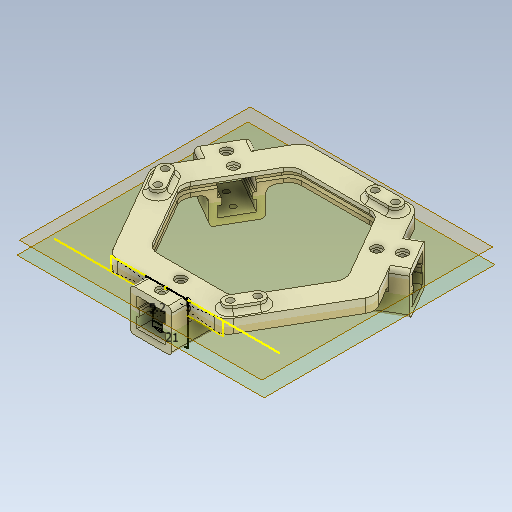
# Autodesk Inventor part: upper_board_mount
Saved by Autodesk Inventor 2021 (Build 250183000, 183)
## iProperties
Created: 2021-01-25
Part Number: upper_board_mount
Material: PC/ABS 플라스틱
Document SubType Name: Modeling
Designer: leejun
Density: 0.357273 g/cm^3
Appearance: 매끄러움 - 물푸레나무색
Author: leejun
Autodesk Inventor part; units mm, degrees
ref_plane "YZ Plane" through (0, 0, 0) normal (1, 0, 0) x (0, 1, 0)
ref_plane "XZ Plane" through (0, 0, 0) normal (0, 1, 0) x (-1, 0, 0)
ref_plane "XY Plane" through (0, 0, 0) normal (0, 0, 1) x (1, 0, 0)
sketch "스케치1" plane through (0, 0, 0) normal (0, 1, 0) x (-1, 0, 0)
  line L0 (128.6603, -74.282) -> (42.8868, -74.282) construction
  line L1 (-128.6603, -74.282) -> (0, 148.5641) construction
  line L2 (0, 148.5641) -> (128.6603, -74.282) construction
  line L3 (40, -69.282) -> (-40, -69.282) construction
  line L4 (-40, -69.282) -> (-40, -56.582) construction
  line L5 (-40, -56.582) -> (40, -56.582) construction
  line L6 (40, -56.582) -> (40, -69.282) construction
  line L7 (-80, 0) -> (-40, 69.282) construction
  line L8 (-40, 69.282) -> (-29.0015, 62.932) construction
  line L9 (-29.0015, 62.932) -> (-69.0015, -6.35) construction
  line L10 (-69.0015, -6.35) -> (-80, 0) construction
  line L11 (40, 69.282) -> (29.0015, 62.932) construction
  line L12 (29.0015, 62.932) -> (69.0015, -6.35) construction
  line L13 (69.0015, -6.35) -> (80, 0) construction
  line L14 (80, 0) -> (40, 69.282) construction
  line L15 (85.7735, 0) -> (42.8868, -74.282) construction
  line L16 (-42.8868, -74.282) -> (-85.7735, 0) construction
  line L17 (42.8868, 74.282) -> (-42.8868, 74.282) construction
  circle A0 centre (72.0007, 1.1551) radius 6.35 construction
  circle A1 centre (64.5007, 14.1455) radius 6.35 construction
  circle A2 centre (-35, -62.932) radius 6.35 construction
  circle A3 centre (-20, -62.932) radius 6.35 construction
  circle A4 centre (-37.0007, 61.7769) radius 6.35 construction
  circle A5 centre (-44.5007, 48.7865) radius 6.35 construction
  circle A6 centre (72.0007, 1.1551) radius 2.65
  circle A7 centre (64.5007, 14.1455) radius 2.65
  circle A8 centre (-20, -62.932) radius 2.65
  circle A9 centre (-35, -62.932) radius 2.65
  circle A10 centre (-44.5007, 48.7865) radius 2.65
  circle A11 centre (-37.0007, 61.7769) radius 2.65
  line L18 (40, -56.582) -> (-40, -69.282) construction
  line L19 (-40, -56.582) -> (40, -69.282) construction
  line L20 (69.0015, -6.35) -> (40, 69.282) construction
  line L21 (80, 0) -> (29.0015, 62.932) construction
  line L22 (-29.0015, 62.932) -> (-80, 0) construction
  line L23 (-69.0015, -6.35) -> (-40, 69.282) construction
  line L24 (72.0007, 1.1551) -> (64.5007, 14.1455) construction
  line L25 (-20, -62.932) -> (-35, -62.932) construction
  line L26 (-37.0007, 61.7769) -> (-44.5007, 48.7865) construction
  circle A12 centre (35, -62.932) radius 2.15 construction
  circle A13 centre (20, -62.932) radius 2.15 construction
  circle A14 centre (44.5007, 48.7865) radius 2.15 construction
  circle A15 centre (37.0007, 61.7769) radius 2.15 construction
  circle A16 centre (-72.0007, 1.1551) radius 2.15 construction
  circle A17 centre (-64.5007, 14.1455) radius 2.15 construction
  line L27 (42.8868, -74.282) -> (-42.8868, -74.282) construction
  line L28 (-42.8868, -74.282) -> (-128.6603, -74.282) construction
  line L29 (0, -62.932) -> (-54.5007, 31.466) construction
  line L30 (-54.5007, 31.466) -> (54.5007, 31.466) construction
  line L31 (54.5007, 31.466) -> (0, -62.932) construction
  line L32 (68.844, -27.6227) -> (58.344, -45.8093)
  line L33 (58.344, -45.8093) -> (40.1575, -35.3093)
  line L34 (40.1575, -35.3093) -> (50.6575, -17.1227)
  line L35 (50.6575, -17.1227) -> (68.844, -27.6227)
  line L36 (10.5, 73.432) -> (-10.5, 73.432)
  line L37 (-10.5, 73.432) -> (-10.5, 52.432)
  line L38 (-10.5, 52.432) -> (10.5, 52.432)
  line L39 (10.5, 52.432) -> (10.5, 73.432)
  line L40 (-58.344, -45.8093) -> (-68.844, -27.6227)
  line L41 (-68.844, -27.6227) -> (-50.6575, -17.1227)
  line L42 (-50.6575, -17.1227) -> (-40.1575, -35.3093)
  line L43 (-40.1575, -35.3093) -> (-58.344, -45.8093)
  line L44 (45.4075, -26.216) -> (-45.4075, -26.216) construction
  line L45 (-45.4075, -26.216) -> (0, 52.432) construction
  line L46 (0, 52.432) -> (45.4075, -26.216) construction
  line L47 (61.8712, 0) -> (30.9356, -53.582)
  line L48 (30.9356, -53.582) -> (-30.9356, -53.582)
  line L49 (-30.9356, -53.582) -> (-61.8712, 0)
  line L50 (-61.8712, 0) -> (-30.9356, 53.582)
  line L51 (-30.9356, 53.582) -> (30.9356, 53.582)
  line L52 (30.9356, 53.582) -> (61.8712, 0)
  line L53 (83.4641, 0) -> (41.7321, -72.282)
  line L54 (41.7321, -72.282) -> (-41.7321, -72.282)
  line L55 (-41.7321, -72.282) -> (-83.4641, 0)
  line L56 (-83.4641, 0) -> (-41.7321, 72.282)
  line L57 (-41.7321, 72.282) -> (41.7321, 72.282)
  line L58 (41.7321, 72.282) -> (83.4641, 0)
  line L59 (68.844, -27.6227) -> (40.1575, -35.3093) construction
  line L60 (58.344, -45.8093) -> (50.6575, -17.1227) construction
  circle A18 centre (54.5007, -31.466) radius 9.35 construction
  line L61 (71.0668, -21.4727) -> (73.9536, -26.4727)
  line L62 (73.9536, -26.4727) -> (59.9029, -50.8093)
  line L63 (59.9029, -50.8093) -> (54.1293, -50.8093)
  line L64 (54.8721, -12.1227) -> (49.0986, -12.1227)
  line L65 (49.0986, -12.1227) -> (35.0479, -36.4593)
  line L66 (35.0479, -36.4593) -> (37.9347, -41.4593)
  line L67 (16.9375, 53.582) -> (14.0507, 48.582)
  line L68 (14.0507, 48.582) -> (-14.0507, 48.582)
  line L69 (-14.0507, 48.582) -> (-16.9375, 53.582)
  line L70 (16.9375, 72.282) -> (14.0507, 77.282)
  line L71 (14.0507, 77.282) -> (-14.0507, 77.282)
  line L72 (-14.0507, 77.282) -> (-16.9375, 72.282)
  line L73 (-37.9347, -41.4593) -> (-35.0479, -36.4593)
  line L74 (-35.0479, -36.4593) -> (-49.0986, -12.1227)
  line L75 (-49.0986, -12.1227) -> (-54.8721, -12.1227)
  line L76 (-71.0668, -21.4727) -> (-73.9536, -26.4727)
  line L77 (-73.9536, -26.4727) -> (-59.9029, -50.8093)
  line L78 (-59.9029, -50.8093) -> (-54.1293, -50.8093)
  line L79 (42.8868, 74.282) -> (40, 69.282) construction
  line L80 (80, 0) -> (85.7735, 0) construction
  point P0 (0, 0)
  point P1 (0, 0)
  point P2 (0, 0)
  point P3 (0, 0)
  point P4 (0, 0)
  point P5 (0, 0)
  point P6 (0, 0)
  dimension "d1" = 12.7
  dimension "d12" = 80
  dimension "d13" = 5.3
  dimension "d14" = 5
  dimension "d15" = 20
  dimension "d16" = 5
  dimension "d17" = 20
  dimension "d18" = 5
  dimension "d19" = 20
  dimension "d79" = 4.3
  dimension "d80" = 5
  dimension "d81" = 15
  dimension "d82" = 5
  dimension "d83" = 15
  dimension "d84" = 5
  dimension "d85" = 15
  dimension "d86" = 5
  dimension "d88" = 21
  dimension "d89" = 3
  dimension "d90" = 3
  dimension "d92" = 5
  dimension "d93" = 5
  dimension "d95" = 5
  dimension "d96" = 5
  dimension "d97" = 5
  dimension "d98" = 5
  dimension "d99" = 5
  dimension "d100" = 5
  dimension "d101" = 5
  dimension "d102" = 5
  dimension "d103" = 5
  dimension "d104" = 5
  dimension "d105" = 5
  dimension "d106" = 5
  dimension "d107" = 5
  dimension "d108" = 5
  dimension "d136" = 5
  dimension "d137" = 5
  constraints: 162 end point, 39 parallel, 24 point on line, 19 centre point, 14 tangent, 13 horizontal, 12 coincident, 12 equal length, 10 equal radius, 7 midpoint, 6 perpendicular, 47 other
  measures "d1" distance of L12.end L13.end
  measures "d12" distance of L11.end L12.end
  measures "d13" diameter of A6
  measures "d14" distance from line of L13 A0.centre
  measures "d15" distance from line of A1.centre L13
  measures "d16" distance from line of L4 A2.centre
  measures "d17" distance from line of L4 A3.centre
  measures "d18" distance from line of L8 A4.centre
  measures "d19" distance from line of L8 A5.centre
  measures "d79" diameter of A12
  measures "d80" distance from line of A12.centre L6
  measures "d81" distance of A13.centre A12.centre
  measures "d82" distance from line of L11 A15.centre
  measures "d83" distance of A15.centre A14.centre
  measures "d84" distance from line of A16.centre L10
  measures "d85" distance of A17.centre A16.centre
  measures "d86" distance between parallel lines of L14 L2
  measures "d88" distance of L33.end L34.end
  measures "d89" distance between parallel lines of L14 L58
  measures "d90" distance between parallel lines of L12 L52
  measures "d92" distance from line of L32.start L61
  measures "d93" distance from line of L63 L32.end
  measures "d95" distance from line of L66 L33.end
  measures "d96" distance from line of L64 L34.end
  measures "d97" distance between parallel lines of L71 L57
  measures "d98" distance from line of L36.start L70
  measures "d99" distance from line of L72 L36.end
  measures "d100" distance between parallel lines of L51 L68
  measures "d101" distance from line of L38.end L67
  measures "d102" distance from line of L37.end L69
  measures "d103" distance between parallel lines of L49 L74
  measures "d104" distance from line of L42.end L73
  measures "d105" distance from line of L75 L41.end
  measures "d106" distance between parallel lines of L77 L55
  measures "d107" distance from line of L40.start L78
  measures "d108" distance from line of L76 L40.end
  measures "d136" distance between parallel lines of L53 L62
  measures "d137" distance between parallel lines of L65 L47
extrude "돌출1" add sketch "스케치1" against normal blind 10 contours L53 L33 L47 L35 | L35 L47 L52 L51 L39 L57 L58 L53 | L53 L54 L55 L43 L49 L48 L47 L33 | L39 L51 L37 L57 | L55 L41 L49 L43 | L37 L51 L50 L49 L41 L55 L56 L57
sketch "스케치2" plane through (0, 0, 0) normal (0, 1, 0) x (1, 0, 0)
  circle A0 centre (37.0007, -61.7769) radius 2.65 projected
  circle A1 centre (44.5007, -48.7865) radius 2.65 projected
  circle A2 centre (20, 62.932) radius 2.65 projected
  circle A3 centre (35, 62.932) radius 2.65 projected
  circle A4 centre (-64.5007, -14.1455) radius 2.65 projected
  circle A5 centre (-72.0007, -1.1551) radius 2.65 projected
  line L0 (37.0007, -61.7769) -> (44.5007, -48.7865) construction
  line L1 (41.3309, -64.2769) -> (48.8309, -51.2865)
  line L2 (40.1706, -46.2865) -> (32.6706, -59.2769)
  arc A6 (32.6706, -59.2769) -> (41.3309, -64.2769) centre (37.0007, -61.7769) ccw
  arc A7 (48.8309, -51.2865) -> (40.1706, -46.2865) centre (44.5007, -48.7865) ccw
  line L3 (-64.5007, -14.1455) -> (-72.0007, -1.1551) construction
  line L4 (-60.1706, -11.6455) -> (-67.6706, 1.3449)
  line L5 (-76.3309, -3.6551) -> (-68.8309, -16.6455)
  arc A8 (-68.8309, -16.6455) -> (-60.1706, -11.6455) centre (-64.5007, -14.1455) ccw
  arc A9 (-67.6706, 1.3449) -> (-76.3309, -3.6551) centre (-72.0007, -1.1551) ccw
  line L6 (20, 62.932) -> (35, 62.932) construction
  line L7 (20, 57.932) -> (35, 57.932)
  line L8 (35, 67.932) -> (20, 67.932)
  arc A10 (20, 67.932) -> (20, 57.932) centre (20, 62.932) ccw
  arc A11 (35, 57.932) -> (35, 67.932) centre (35, 62.932) ccw
  point P0 (0, 0)
  point P1 (40.7507, -55.2817)
  point P2 (-68.2507, -7.6503)
  point P3 (27.5, 62.932)
  dimension "d26" = 5
  constraints: 24 end point, 12 point on circle, 12 tangent, 6 centre point, 3 midpoint, 3 parallel, 2 equal radius, 1 horizontal
  measures "d26" radius of A6
extrude "돌출2" add sketch "스케치2" along normal blind 5 contours A0 | A1 | A2 | A3 | A4 | A5 | A6 L2 A7 L1 | A8 L5 A9 L4 | A10 L8 A11 L7
extrude "돌출3" cut sketch "스케치2" along normal through all both and the other way through all contours A0 | A1 | A2 | A3 | A4 | A5
fillet "모깎기1" radius 3 12 edges at (-74.5007, 0, -3.175) (-63.9206, 0, 5.1503) (-62.0007, 0, 18.4756) (-72.5809, 0, 10.1503) (36.4206, 0, 52.7817) (47.0007, 0, 44.4564) (45.0809, 0, 57.7817) (34.5007, 0, 66.107) (27.5, 0, -67.932) (40, 0, -62.932) (27.5, 0, -57.932) (15, 0, -62.932)
sketch "스케치9" plane through (0, -10, 0) normal (0, -1, 0) x (1, 0, 0)
  circle A0 centre (35, -62.932) radius 2.65 projected
  circle A1 centre (20, -62.932) radius 2.65 projected
  circle A2 centre (44.5007, 48.7865) radius 2.65 projected
  circle A3 centre (37.0007, 61.7769) radius 2.65 projected
  circle A4 centre (-64.5007, 14.1455) radius 2.65 projected
  circle A5 centre (-72.0007, 1.1551) radius 2.65 projected
  circle A6 centre (35, -62.932) radius 4.4
  circle A7 centre (20, -62.932) radius 4.4
  circle A8 centre (44.5007, 48.7865) radius 2.65 projected
  circle A9 centre (44.5007, 48.7865) radius 4.4
  circle A10 centre (37.0007, 61.7769) radius 2.65 projected
  circle A11 centre (37.0007, 61.7769) radius 4.4
  circle A12 centre (-64.5007, 14.1455) radius 4.4
  circle A13 centre (-72.0007, 1.1551) radius 4.4
  point P0 (0, 0)
  dimension "d65" = 8.8
  constraints: 6 centre point, 6 coincident, 5 equal radius
  measures "d65" diameter of A6
extrude "돌출11" cut sketch "스케치9" against normal blind 3 contours A0 | A1 | A2 | A3 | A4 | A5 | A6 | A7 | A9 | A11 | A12 | A13
sketch "스케치15" plane through (-41.7321, 0, 72.282) normal (0, 0, 1) x (1, 0, 0)
  line L0 (0, 0) -> (83.4641, 0) projected
  line L1 (0, 0) -> (0, -10) projected
  line L2 (83.4641, -10) -> (0, -10) projected
  line L3 (83.4641, 0) -> (83.4641, -10) projected
  line L4 (0, -10) -> (-41.7321, -10) projected
  line L5 (125.1962, 0) -> (83.4641, 0) projected
  line L6 (0, -10) -> (83.4641, 0) construction
  line L7 (0, 0) -> (0, -10) projected
  line L8 (0, 0) -> (83.4641, -10) construction
  line L9 (31.2321, -26) -> (52.2321, -26)
  line L10 (52.2321, -26) -> (52.2321, -5)
  line L11 (52.2321, -5) -> (31.2321, -5)
  line L12 (31.2321, -5) -> (31.2321, -26)
  line L13 (31.2321, -26) -> (52.2321, -5) construction
  line L14 (52.2321, -26) -> (31.2321, -5) construction
  line L15 (57.2321, 0) -> (57.2321, -31)
  line L16 (57.2321, -31) -> (26.2321, -31)
  line L17 (26.2321, -31) -> (26.2321, 0)
  line L18 (26.2321, 0) -> (57.2321, 0)
  line L19 (0, 0) -> (83.4641, 0) projected
  line L20 (31.2321, -18.1) -> (33.2321, -18.1)
  line L21 (33.2321, -18.1) -> (33.2321, -12.9)
  line L22 (33.2321, -12.9) -> (31.2321, -12.9)
  line L23 (31.2321, -12.9) -> (31.2321, -18.1)
  line L24 (31.2321, -18.1) -> (33.2321, -12.9) construction
  line L25 (33.2321, -18.1) -> (31.2321, -12.9) construction
  line L26 (50.2321, -18.1) -> (52.2321, -18.1)
  line L27 (52.2321, -18.1) -> (52.2321, -12.9)
  line L28 (52.2321, -12.9) -> (50.2321, -12.9)
  line L29 (50.2321, -12.9) -> (50.2321, -18.1)
  line L30 (50.2321, -18.1) -> (52.2321, -12.9) construction
  line L31 (52.2321, -18.1) -> (50.2321, -12.9) construction
  point P0 (41.7321, 0)
  point P1 (41.7321, -15.5)
  point P2 (41.7321, -5)
  point P3 (41.7321, -15.5)
  point P4 (32.2321, -15.5)
  point P5 (51.2321, -15.5)
  point P6 (32.2321, -15.5)
  point P7 (41.7321, -15.5)
  point P8 (51.2321, -15.5)
  point P9 (39.0956, -5)
  point P10 (31.2321, -10)
  point P11 (52.2321, -10)
  point P12 (44.2956, -5)
  point P13 (57.2321, -10)
  point P14 (44.3321, -26)
  point P15 (39.1321, -26)
  point P16 (26.2321, -10)
  point P17 (32.2321, -15.5)
  point P18 (51.2321, -15.5)
  point P19 (31.2321, -18.1)
  point P20 (31.2321, -12.9)
  dimension "d140" = 21
  dimension "d141" = 5
  dimension "d142" = 2
  dimension "d143" = 5.2
  constraints: 48 end point, 13 midpoint, 8 parallel, 4 perpendicular, 3 collinear, 3 equal length, 3 horizontal, 2 horizontal alignment, 1 vertical alignment, 3 other
  measures "d140" distance of L9.start L9.end
  measures "d141" distance between parallel lines of L11 L0
  measures "d142" distance of L20.start L20.end
  measures "d143" distance of L20.end L21.end
extrude "돌출18" cut sketch "스케치15" against normal up to surface (18.7 mm away) contours L12 L11 L10 L2
extrude "돌출19" add sketch "스케치15" against normal up to surface (18.7 mm away) contours L0 L15 L2 L10 L11 L12 L17 | L2 L12 L9 L10 L15 L16 L17 | L22 L21 L20 L12 | L10 L26 L29 L28
extrude "돌출20" add sketch "스케치15" along normal blind 11.3 contours L0 L15 L2 L10 L11 L12 L17 | L2 L12 L9 L10 L15 L16 L17 | L22 L21 L20 L12 | L10 L26 L29 L28
sketch "스케치20" plane through (-15.5, -31, 53.582) normal (0, -1, 0) x (1, 0, 0)
  line L0 (26, 0) -> (5, 0) projected
  line L1 (5, 0) -> (5, 30) projected
  line L2 (26, 30) -> (5, 30) projected
  line L3 (26, 0) -> (26, 30) projected
  circle A0 centre (15.5, 22) radius 10.5 construction
  circle A1 centre (15.5, 8) radius 2.1
  circle A2 centre (15.5, 22) radius 2.1
  circle A3 centre (15.5, 22) radius 3.9
  circle A4 centre (15.5, 8) radius 3.9
  point P0 (15.5, -53.582)
  dimension "d188" = 8
  dimension "d189" = 8
  dimension "d190" = 4.2
  dimension "d191" = 7.8
  constraints: 5 centre point, 3 coincident, 2 equal radius, 2 tangent, 1 vertical alignment
  measures "d188" distance from line of L0 A1.centre
  measures "d189" distance from line of L2 A2.centre
  measures "d190" diameter of A1
  measures "d191" diameter of A3
extrude "돌출25" cut sketch "스케치20" against normal through all contours A1 | A2
extrude "돌출26" cut sketch "스케치20" against normal blind 2 contours A3 | A4
ref_plane "작업 평면15" through (-10.5, -15.5, 53.582) normal (0, -1, 0) x (1, 0, 0)
mirror "미러6" about plane through (-10.5, -15.5, 53.582) normal (0, -1, 0) of "돌출26"
pattern_circular "원형 패턴6" count 3 over 360 about axis through (0, -10, 0) along (0, 1, 0) of "돌출26", "미러6", "돌출25", "돌출20", "돌출19", "돌출18"
fillet "모깎기5" radius 10 12 edges at (-83.4641, -5, 0) (-41.7321, -5, 72.282) (41.7321, -5, 72.282) (83.4641, -5, 0) (41.7321, -5, -72.282) (-41.7321, -5, -72.282) (-61.8712, -5, 0) (-30.9356, -5, -53.582) (30.9356, -5, -53.582) (61.8712, -5, 0) (30.9356, -5, 53.582) (-30.9356, -5, 53.582)
fillet "모깎기5" radius 3 12 edges at (-51.6438, -31, -47.7144) (-67.1438, -31, -20.8676) (-59.7411, 0, -52.3894) (-75.2411, 0, -25.5426) (-15.5, 0, 77.932) (15.5, 0, 77.932) (-15.5, -31, 68.582) (15.5, -31, 68.582) (67.1438, -31, -20.8676) (51.6438, -31, -47.7144) (75.2411, 0, -25.5426) (59.7411, 0, -52.3894)
fillet "모깎기5" radius 1 12 edges at (55.1438, -18.1, -41.6522) (55.1438, -12.9, -41.6522) (63.6438, -12.9, -26.9298) (63.6438, -18.1, -26.9298) (-63.6438, -18.1, -26.9298) (-63.6438, -12.9, -26.9298) (-55.1438, -12.9, -41.6522) (-55.1438, -18.1, -41.6522) (-8.5, -18.1, 68.582) (8.5, -18.1, 68.582) (8.5, -12.9, 68.582) (-8.5, -12.9, 68.582)
fillet "모깎기5" radius 5 6 edges at (46.7507, -10, -44.8894) (-46.7507, -10, -44.8894) (-62.2507, -10, -18.0426) (-15.5, -10, 62.932) (62.2507, -10, -18.0426) (15.5, -10, 62.932)
ref_plane "작업 평면16" through (0, -5, 0) normal (0, 1, 0) x (1, 0, 0)
sketch "스케치21" plane through (0, -5, 0) normal (0, 1, 0) x (1, 0, 0)
  line L0 (-50.4696, 31.4481) -> (-56.5318, 34.9481) projected
  line L1 (-56.5318, 34.9481) -> (-55.0318, 37.5461) projected
  line L2 (-55.0318, 37.5461) -> (-48.9696, 34.0461) projected
  line L3 (-48.9696, 34.0461) -> (-50.4696, 31.4481) projected
  line L4 (50.4696, -31.4481) -> (56.5318, -34.9481) projected
  line L5 (56.5318, -34.9481) -> (55.0318, -37.5461) projected
  line L6 (55.0318, -37.5461) -> (48.9696, -34.0461) projected
  line L7 (48.9696, -34.0461) -> (50.4696, -31.4481) projected
  line L8 (-43.4696, 43.5724) -> (-49.5318, 47.0724) projected
  line L9 (-49.5318, 47.0724) -> (-48.0318, 49.6705) projected
  line L10 (-48.0318, 49.6705) -> (-41.9696, 46.1705) projected
  line L11 (-41.9696, 46.1705) -> (-43.4696, 43.5724) projected
  line L12 (48.0318, -49.6705) -> (41.9696, -46.1705) projected
  line L13 (41.9696, -46.1705) -> (43.4696, -43.5724) projected
  line L14 (43.4696, -43.5724) -> (49.5318, -47.0724) projected
  line L15 (49.5318, -47.0724) -> (48.0318, -49.6705) projected
  circle A0 centre (-49.5007, 40.1263) radius 2.1 projected
  circle A1 centre (49.5007, -40.1263) radius 2.1 projected
  circle A2 centre (-42.0007, 53.1167) radius 2.1 projected
  circle A3 centre (42.0007, -53.1167) radius 2.1 projected
  circle A4 centre (-44.5007, -48.7865) radius 3.9 projected
  circle A5 centre (-37.0007, -61.7769) radius 3.9 projected
  circle A6 centre (-20, 62.932) radius 3.9 projected
  circle A7 centre (-35, 62.932) radius 3.9 projected
  circle A8 centre (64.5007, -14.1455) radius 3.9 projected
  circle A9 centre (72.0007, -1.1551) radius 3.9 projected
  arc A10 (-35.9585, 72.282) -> (-44.6188, 67.282) centre (-35.9585, 62.282) ccw projected
  line L16 (-44.6188, 67.282) -> (-80.5774, 5) projected
  arc A11 (-80.5774, 5) -> (-80.5774, -5) centre (-71.9171, 0) ccw projected
  line L17 (-80.5774, -5) -> (-44.6188, -67.282) projected
  arc A12 (-44.6188, -67.282) -> (-35.9585, -72.282) centre (-35.9585, -62.282) ccw projected
  line L18 (-35.9585, -72.282) -> (35.9585, -72.282) projected
  arc A13 (35.9585, -72.282) -> (44.6188, -67.282) centre (35.9585, -62.282) ccw projected
  line L19 (44.6188, -67.282) -> (80.5774, -5) projected
  arc A14 (80.5774, -5) -> (80.5774, 5) centre (71.9171, 0) ccw projected
  line L20 (80.5774, 5) -> (44.6188, 67.282) projected
  arc A15 (44.6188, 67.282) -> (35.9585, 72.282) centre (35.9585, 62.282) ccw projected
  line L21 (35.9585, 72.282) -> (-35.9585, 72.282) projected
  line L22 (33.8224, 48.582) -> (58.9845, 5) projected
  arc A16 (58.9845, -5) -> (58.9845, 5) centre (50.3242, 0) ccw projected
  line L23 (58.9845, -5) -> (33.8224, -48.582) projected
  arc A17 (25.1621, -53.582) -> (33.8224, -48.582) centre (25.1621, -43.582) ccw projected
  line L24 (25.1621, -53.582) -> (-25.1621, -53.582) projected
  arc A18 (-33.8224, -48.582) -> (-25.1621, -53.582) centre (-25.1621, -43.582) ccw projected
  line L25 (-33.8224, -48.582) -> (-58.9845, -5) projected
  arc A19 (-58.9845, 5) -> (-58.9845, -5) centre (-50.3242, 0) ccw projected
  line L26 (-58.9845, 5) -> (-33.8224, 48.582) projected
  arc A20 (-25.1621, 53.582) -> (-33.8224, 48.582) centre (-25.1621, 43.582) ccw projected
  line L27 (-25.1621, 53.582) -> (25.1621, 53.582) projected
  arc A21 (33.8224, 48.582) -> (25.1621, 53.582) centre (25.1621, 43.582) ccw projected
  line L28 (25.1621, 56.582) -> (-25.1621, 56.582)
  arc A22 (-25.1621, 56.582) -> (-36.4204, 50.082) centre (-25.1621, 43.582) ccw
  line L29 (-36.4204, 50.082) -> (-61.5825, 6.5)
  arc A23 (-61.5825, 6.5) -> (-61.5825, -6.5) centre (-50.3242, 0) ccw
  line L30 (-61.5825, -6.5) -> (-36.4204, -50.082)
  arc A24 (-36.4204, -50.082) -> (-25.1621, -56.582) centre (-25.1621, -43.582) ccw
  line L31 (-25.1621, -56.582) -> (25.1621, -56.582)
  arc A25 (25.1621, -56.582) -> (36.4204, -50.082) centre (25.1621, -43.582) ccw
  line L32 (36.4204, -50.082) -> (61.5825, -6.5)
  arc A26 (61.5825, -6.5) -> (61.5825, 6.5) centre (50.3242, 0) ccw
  line L33 (61.5825, 6.5) -> (36.4204, 50.082)
  arc A27 (36.4204, 50.082) -> (25.1621, 56.582) centre (25.1621, 43.582) ccw
  point P0 (0, 0)
  dimension "d203" = 3
  constraints: 12 end point, 12 point on circle, 6 centre point, 11 other
  measures "d203" distance between parallel lines of L27 L28
extrude "돌출27" cut sketch "스케치21" along normal mid plane 4 contours A27 L33 A26 L32 A25 L31 A24 L30 A23 L29 A22 L28
equation "\"d16\" = d14"
equation "\"d17\" = d15"
equation "\"d18\" = d14"
equation "\"d19\" = d15"
